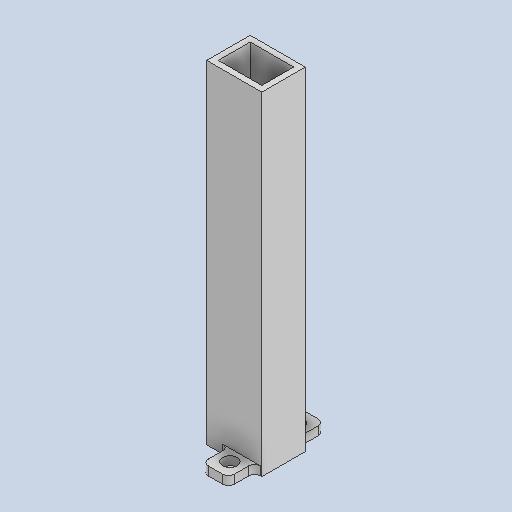
# Autodesk Inventor part: neck
Saved by Autodesk Inventor 2025 (Build 290162000, 162)
## iProperties
Created: 2025-09-04
Part Number: neck
Material: Generic
Document SubType Name: Modeling
Designer: Pravoslav
Density: 1 g/cm^3
Appearance: Default
Author: Pravoslav
Autodesk Inventor part; units mm, degrees
ref_plane "YZ Plane" through (0, 0, 0) normal (1, 0, 0) x (0, 1, 0)
ref_plane "XZ Plane" through (0, 0, 0) normal (0, 1, 0) x (-1, 0, 0)
ref_plane "XY Plane" through (0, 0, 0) normal (0, 0, 1) x (1, 0, 0)
sketch "Sketch1" plane through (0, 0, 0) normal (0, 1, 0) x (-1, 0, 0)
  line L0 (9.5, 7.5) -> (-9.5, 7.5)
  line L1 (-9.5, 7.5) -> (-9.5, -7.5)
  line L2 (-9.5, -7.5) -> (9.5, -7.5)
  line L3 (9.5, -7.5) -> (9.5, 7.5)
  line L4 (9.5, 7.5) -> (-9.5, -7.5) construction
  line L5 (-9.5, 7.5) -> (9.5, -7.5) construction
  line L6 (7.5, 5.5) -> (-7.5, 5.5)
  line L7 (-7.5, 5.5) -> (-7.5, -5.5)
  line L8 (-7.5, -5.5) -> (7.5, -5.5)
  line L9 (7.5, -5.5) -> (7.5, 5.5)
  line L10 (7.5, 5.5) -> (-7.5, -5.5) construction
  line L11 (-7.5, 5.5) -> (7.5, -5.5) construction
  point P0 (0, 0)
  dimension "d0" = 19
  dimension "d1" = 15
  dimension "d2" = 2
  dimension "d3" = 2
  constraints: 24 end point, 4 midpoint, 4 parallel, 2 horizontal, 2 perpendicular
  measures "d0" distance of L2.end L1.end
  measures "d1" distance of L1.end L0.end
  measures "d2" distance between parallel lines of L3 L9
  measures "d3" distance between parallel lines of L2 L8
extrude "Extrusion1" add sketch "Sketch1" along normal blind 115
sketch "Sketch3" plane through (0, 0, 0) normal (0, -1, 0) x (1, 0, 0)
  circle A0 centre (2.5, 11.5) radius 2.5
  circle A1 centre (2.5, -11.5) radius 2.5
  line L0 (-9.5, -7.5) -> (-9.5, 7.5) projected
  line L1 (-9.5, 7.5) -> (9.5, 7.5) projected
  line L2 (-2, 7.5) -> (7, 7.5)
  line L3 (7, 7.5) -> (7, 16.5)
  line L4 (7, 16.5) -> (-2, 16.5)
  line L5 (-2, 16.5) -> (-2, 7.5)
  line L6 (0, 0) -> (7.5, 0)
  line L7 (7.5, -5.5) -> (7.5, 5.5) projected
  circle A2 centre (2.5, -11.5) radius 2.5
  line L8 (-9.5, -7.5) -> (9.5, -7.5)
  line L9 (7, -7.5) -> (7, -16.5)
  line L10 (7, -16.5) -> (-2, -16.5)
  line L11 (-2, -16.5) -> (-2, -7.5)
  dimension "d13" = 5
  dimension "d14" = 5
  dimension "d15" = 23
  dimension "d16" = 11.5
  dimension "d17" = 12
  dimension "d18" = 12
  dimension "d19" = 9
  dimension "d20" = 9
  dimension "d21" = 4.5
  constraints: 18 end point, 6 symmetric about line, 3 centre point, 2 parallel, 2 point on line, 1 horizontal, 1 midpoint, 1 perpendicular, 1 other
  measures "d13" diameter of A0
  measures "d14" diameter of A1
  measures "d15" distance of A1.centre A0.centre
  measures "d16" vertical distance of L6.start A1.centre
  measures "d17" distance from line of L0 A0.centre
  measures "d18" distance from line of L0 A1.centre
  measures "d19" distance between parallel lines of L5 L3
  measures "d20" distance between parallel lines of L1 L4
  measures "d21" distance from line of A0.centre L3
extrude "Extrusion3" add sketch "Sketch3" against normal blind 3
fillet "Fillet2" radius 2 8 edges at (-2, 1.5, -7.5) (-2, 1.5, -16.5) (7, 1.5, -16.5) (7, 1.5, -7.5) (7, 1.5, 7.5) (7, 1.5, 16.5) (-2, 1.5, 16.5) (-2, 1.5, 7.5)
sketch "Sketch2" plane through (0, 0, 0) normal (0, -1, 0) x (1, 0, 0)
  circle A0 centre (-11.5, 0) radius 2.5
  circle A1 centre (11.5, 0) radius 2.5
  line L0 (-14.8361, 4.3238) -> (-8.1639, 4.3238)
  line L1 (-8.1639, 4.3238) -> (-8.1639, -4.3238)
  line L2 (-8.1639, -4.3238) -> (-14.8361, -4.3238)
  line L3 (-14.8361, -4.3238) -> (-14.8361, 4.3238)
  line L4 (-14.8361, 4.3238) -> (-8.1639, -4.3238) construction
  line L5 (-8.1639, 4.3238) -> (-14.8361, -4.3238) construction
  line L6 (0, 0) -> (0, 5.5)
  line L7 (7.5, 5.5) -> (-7.5, 5.5) projected
  line L8 (14.8361, 4.3238) -> (8.1639, 4.3238)
  line L9 (8.1639, 4.3238) -> (8.1639, -4.3238)
  line L10 (8.1639, -4.3238) -> (14.8361, -4.3238)
  line L11 (14.8361, -4.3238) -> (14.8361, 4.3238)
  dimension "d6" = 5
  dimension "d7" = 5
  dimension "d8" = 23
  dimension "d9" = 11.5
  constraints: 22 end point, 4 symmetric about line, 3 midpoint, 2 centre point, 2 parallel, 1 horizontal, 1 perpendicular
  measures "d6" diameter of A0
  measures "d7" diameter of A1
  measures "d8" distance of A1.centre A0.centre
  measures "d9" distance of L6.start A1.centre
body "Solid1"
